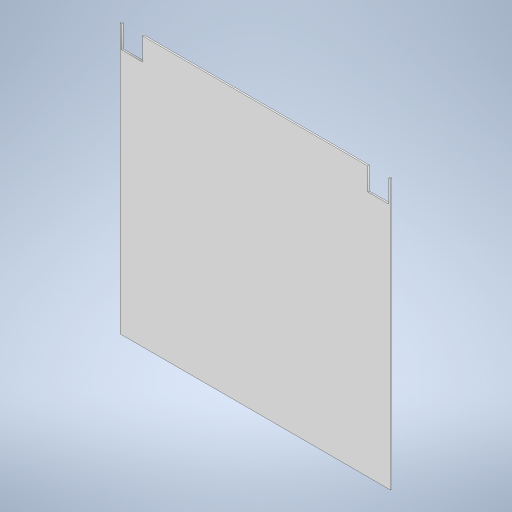
# Autodesk Inventor part: plate_back
Saved by Autodesk Inventor 2023 (Build 270158000, 158)
## iProperties
Created: 2023-08-22
Part Number: plate_back
Material: Polystyrene
Document SubType Name: Modeling
Designer: chriboehm
Density: 1.021 g/cm^3
Appearance: White
Author: chriboehm
Autodesk Inventor part; units mm, degrees
ref_plane "YZ Plane" through (0, 0, 0) normal (1, 0, 0) x (0, 1, 0)
ref_plane "XZ Plane" through (0, 0, 0) normal (0, 1, 0) x (-1, 0, 0)
ref_plane "XY Plane" through (0, 0, 0) normal (0, 0, 1) x (1, 0, 0)
sketch "Sketch1" plane through (0, 0, 0) normal (0, 0, 1) x (1, 0, 0)
  line L0 (0, 0) -> (542, 0)
  line L1 (542, 0) -> (542, 495)
  line L2 (497, 540) -> (45, 540)
  line L3 (0, 495) -> (0, 0)
  line L4 (45, 540) -> (45, 495)
  line L5 (45, 495) -> (0, 495)
  line L6 (497, 540) -> (497, 495)
  line L7 (497, 495) -> (542, 495)
  line L8 (0, 495) -> (3, 495)
  line L9 (3, 495) -> (3, 540)
  line L10 (3, 540) -> (0, 540)
  line L11 (0, 540) -> (0, 495)
  line L12 (542, 495) -> (539, 495)
  line L13 (539, 495) -> (539, 540)
  line L14 (539, 540) -> (542, 540)
  line L15 (542, 540) -> (542, 495)
  dimension "d0" = 542
  dimension "d1" = 540
  dimension "d4" = 45
  dimension "d5" = 45
  dimension "d6" = 45
  dimension "d7" = 45
  dimension "d8" = 3
  dimension "d9" = 3
  constraints: 32 end point, 6 parallel, 5 perpendicular, 3 horizontal, 2 vertical
  measures "d0" distance of L1.end L3.start
  measures "d1" distance between parallel lines of L0 L2
  measures "d4" distance between parallel lines of L3 L4
  measures "d5" distance between parallel lines of L2 L5
  measures "d6" distance between parallel lines of L2 L7
  measures "d7" distance between parallel lines of L1 L6
  measures "d8" distance between parallel lines of L11 L9
  measures "d9" distance between parallel lines of L15 L13
extrude "Extrusion1" add sketch "Sketch1" along normal blind 3
equation "\"d5\" = d4"
equation "\"d6\" = d5"
equation "\"d7\" = d6"
body "Solid1"
